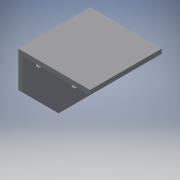
# Autodesk Inventor part: angle gusset
Saved by Autodesk Inventor 2016 (Build 200138000, 138)
## iProperties
Created: 2016-02-03
Part Number: angle gusset
Material: Generic
Document SubType Name: Modeling
Designer: gus
Density: 1 g/cm^3
Appearance: Default
Author: gus
Autodesk Inventor part; units mm, degrees
ref_plane "YZ Plane" through (0, 0, 0) normal (1, 0, 0) x (0, 1, 0)
ref_plane "XZ Plane" through (0, 0, 0) normal (0, 1, 0) x (-1, 0, 0)
ref_plane "XY Plane" through (0, 0, 0) normal (0, 0, 1) x (1, 0, 0)
sketch "Sketch1" plane through (0, 0, 0) normal (0, 0, 1) x (1, 0, 0)
  line L0 (0, 0) -> (50.8, 0)
  line L1 (50.8, 0) -> (50.8, -3.175)
  line L2 (50.8, -3.175) -> (3.175, -3.175)
  line L3 (3.175, -3.175) -> (3.175, -50.8)
  line L4 (3.175, -50.8) -> (0, -50.8)
  line L5 (0, -50.8) -> (0, 0)
  dimension "d0" = 50.8
  dimension "d1" = 3.175
  dimension "d2" = 47.625
  dimension "d3" = 47.625
  constraints: 12 end point, 4 perpendicular, 1 horizontal, 1 parallel
  measures "d0" distance of L0.start L0.end
  measures "d1" distance of L0.end L1.end
  measures "d2" distance of L1.end L2.end
  measures "d3" distance of L2.end L3.end
extrude "Extrusion1" add sketch "Sketch1" along normal blind 50.8
sketch "Sketch2" plane through (3.175, -50.8, 0) normal (1, 0, 0) x (0, 0, -1)
  line L0 (-50.8, 50.8) -> (-50.8, 0) projected
  line L1 (-50.8, 25.4) -> (-25.4, 0)
  line L2 (0, 0) -> (-50.8, 0) projected
  line L3 (0, 50.8) -> (-50.8, 50.8) projected
  line L4 (-50.8, 25.4) -> (-50.8, 0)
  line L5 (-25.4, 0) -> (-50.8, 0)
  circle A0 centre (-12.7, 12.7) radius 3.3734
  circle A1 centre (-12.7, 38.1) radius 3.3734
  line L6 (0, 47.625) -> (0, 0) projected
  dimension "d6" = 25.4
  dimension "d12" = 12.7
  dimension "d13" = 12.7
  dimension "d14" = 25.4
  dimension "d15" = 12.7
  dimension "d20" = 6.7469
  dimension "d21" = 6.7469
  constraints: 6 end point, 2 centre point, 2 collinear, 2 midpoint
  measures "d6" distance from line of L3 L1.start
  measures "d12" distance from line of L2 A0.centre
  measures "d13" distance from line of L6 A0.centre
  measures "d14" distance of A0.centre A1.centre
  measures "d15" distance from line of L6 A1.centre
  measures "d20" diameter of A0
  measures "d21" diameter of A1
extrude "Extrusion3" cut sketch "Sketch2" against normal blind 3.175
sketch "Sketch3" plane through (3.175, -3.175, 0) normal (0, -1, 0) x (1, 0, 0)
  circle A0 centre (9.525, 38.1) radius 3.3734
  circle A1 centre (34.925, 12.7) radius 3.3734
  line L0 (47.625, 0) -> (0, 0) projected
  line L1 (47.625, 0) -> (47.625, 50.8) projected
  line L2 (0, 50.8) -> (47.625, 50.8) projected
  line L3 (0, 0) -> (0, 50.8) projected
  point P0 (-3.175, 0)
  dimension "d22" = 6.7469
  dimension "d23" = 6.7469
  dimension "d24" = 12.7
  dimension "d25" = 12.7
  dimension "d26" = 12.7
  dimension "d27" = 9.525
  constraints: 2 centre point
  measures "d22" diameter of A0
  measures "d23" diameter of A1
  measures "d24" distance from line of L0 A1.centre
  measures "d25" distance from line of L1 A1.centre
  measures "d26" distance from line of L2 A0.centre
  measures "d27" distance from line of L3 A0.centre
extrude "Extrusion4" cut sketch "Sketch3" against normal blind 3.175 contours A0 | A1
body "Solid1"
